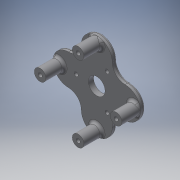
# Autodesk Inventor part: cycloid_motor_fix_plate
Saved by Autodesk Inventor 2019.4 (Build 234330000, 330)
## iProperties
Created: 2019-08-28
Part Number: cycloid_motor_fix_plate
Material: Generic
Document SubType Name: Modeling
Designer: cdi
Density: 1 g/cm^3
Appearance: Default
Author: cdi
Autodesk Inventor part; units mm, degrees
ref_plane "YZ Plane" through (0, 0, 0) normal (1, 0, 0) x (0, 1, 0)
ref_plane "XZ Plane" through (0, 0, 0) normal (0, 1, 0) x (-1, 0, 0)
ref_plane "XY Plane" through (0, 0, 0) normal (0, 0, 1) x (1, 0, 0)
sketch "Sketch1" plane through (0, 0, 0) normal (0, 0, 1) x (1, 0, 0)
  circle A0 centre (0, 0) radius 34
  dimension "d2" = 68
  constraints: 1 centre point, 1 coincident
  measures "d2" diameter of A0
extrude "Extrusion1" add sketch "Sketch1" along normal blind 4
sketch "Sketch3" plane through (0, 0, 0) normal (0, 0, -1) x (-1, 0, 0)
  circle A0 centre (0, 0) radius 6.5
  dimension "d15" = 13
  constraints: 1 centre point, 1 coincident
  measures "d15" diameter of A0
extrude "Extrusion2" cut sketch "Sketch3" against normal through all
sketch "Sketch4" plane through (0, 0, 0) normal (0, 0, -1) x (-1, 0, 0)
  circle A0 centre (0, 0) radius 9.5
  circle A1 centre (0, 9.5) radius 1.5
  circle A2 centre (-6.7175, 6.7175) radius 1.5
  circle A3 centre (-9.5, 0) radius 1.5
  circle A4 centre (-6.7175, -6.7175) radius 1.5
  circle A5 centre (0, -9.5) radius 1.5
  circle A6 centre (6.7175, -6.7175) radius 1.5
  circle A7 centre (9.5, 0) radius 1.5
  circle A8 centre (6.7175, 6.7175) radius 1.5
  circle A9 centre (0, 0) radius 16
  circle A10 centre (16, 0) radius 1.5
  circle A11 centre (-8, 13.8564) radius 1.5
  circle A12 centre (-8, -13.8564) radius 1.5
  point P0 (-6.9376, -6.7295)
  dimension "d18" = 19
  dimension "d24" = 32
  dimension "d19" = 3
  dimension "d22" = 360
  dimension "d25" = 3
  dimension "d28" = 360
  constraints: 11 centre point, 2 coincident, 1 horizontal alignment, 1 vertical alignment, 28 other
  measures "d19" diameter of A1
  measures "d25" diameter of A10
hole "Hole2" at (8, 13.8564, 0) at (-16, 0, 0) at (8, -13.8564, 0) direction (0, 0, 1) diameter 3.1 depth 10 countersink diameter 6.5 countersink angle 90
sketch "Sketch5" plane through (0, 0, 4) normal (0, 0, 1) x (1, 0, 0)
  line L0 (-80.396, -12) -> (-12, -12)
  line L1 (-12, -12) -> (-12, -63.9802)
  line L2 (-12, -63.9802) -> (-80.396, -63.9802)
  line L3 (-80.396, -63.9802) -> (-80.396, -12)
  line L4 (0, 0) -> (-93.0099, 0)
  line L5 (0, 0) -> (0, -83.9307)
  dimension "d37" = 12
  dimension "d38" = 12
  constraints: 12 end point, 2 horizontal, 2 parallel, 1 perpendicular, 1 vertical
  measures "d37" distance between parallel lines of L1 L5
  measures "d38" distance between parallel lines of L4 L0
extrude "Extrusion3" cut sketch "Sketch5" against normal through all
pattern_circular "Circular Pattern2" count 4 over 360 about axis through (0, 0, 0) along (0, 0, 1) of "Extrusion3"
fillet "Fillet1" radius 10 4 edges at (-12, -12, 2) (12, 12, 2) (-12, 12, 2) (12, -12, 2)
fillet "Fillet1" radius 12 8 edges at (12, 31.8119, 2) (-12, 31.8119, 2) (-31.8119, 12, 2) (-31.8119, -12, 2) (-12, -31.8119, 2) (12, -31.8119, 2) (31.8119, -12, 2) (31.8119, 12, 2)
sketch "Sketch6" plane through (0, 0, 4) normal (0, 0, 1) x (1, 0, 0)
  circle A0 centre (0, 29.5) radius 1.625 projected
  circle A1 centre (0, 29.5) radius 4.5
  point P0 (0, 0)
  dimension "d46" = 9
  constraints: 1 centre point, 1 coincident
  measures "d46" diameter of A1
extrude "Extrusion4" add sketch "Sketch6" along normal blind 14.5
pattern_circular "Circular Pattern3" count 4 over 360 about axis through (0, 0, 0) along (0, 0, 1) of "Extrusion4"
fillet "Fillet3" radius 2 12 edges at (-3.1819, 26.318, 4) (3.182, 32.6819, 4) (0, 34, 4) (-26.318, -3.1819, 4) (-32.6819, 3.182, 4) (-34, 0, 4) (3.1819, -26.318, 4) (-3.182, -32.6819, 4) (0, -34, 4) (32.6819, -3.182, 4) (34, 0, 4) (26.318, 3.1819, 4)
fillet "Fillet4" radius 2 24 edges at (-12, -22, 0) (-14.9289, -14.9289, 0) (-22, -12, 0) (12, -22, 0) (8.4853, -30.4853, 0) (-8.4853, -30.4853, 0) (0, -34, 0) (22, -12, 0) (14.9289, -14.9289, 0) (30.4853, 8.4853, 0) (22, 12, 0) (30.4853, -8.4853, 0) (34, 0, 0) (12, 22, 0) (14.9289, 14.9289, 0) (-12, 22, 0) (-8.4853, 30.4853, 0) (8.4853, 30.4853, 0) (0, 34, 0) (-22, 12, 0) (-14.9289, 14.9289, 0) (-30.4853, 8.4853, 0) (-30.4853, -8.4853, 0) (-34, 0, 0)
sketch "Sketch2" plane through (0, 0, 0) normal (0, 0, -1) x (-1, 0, 0)
  circle A0 centre (0, 29.5) radius 3.5
  point P0 (0, 0)
  dimension "d3" = 7
  dimension "d4" = 29.5
  constraints: 1 centre point
  measures "d3" diameter of A0
  measures "d4" distance of point (0, 0) A0.centre
extrude "Extrusion5" cut sketch "Sketch2" against normal blind 3
sketch "Sketch9" plane through (0, 29.5, 3) normal (0, 0, -1) x (-1, 0, 0)
  arc A0 (-2.8, 2.1) -> (2.8, 2.1) centre (0, 0) ccw projected
  point P0 (0, -29.5)
hole "Hole5" at (0, 29.5, 3) direction (0, 0, 1) diameter 3.25 depth 15 countersink diameter 6.5 countersink angle 90
fillet "Fillet6" radius 0.4 5 edges at (1.5811, 32.6225, 0.1417) (-1.5811, 32.6225, 0.1417) (0, 33, 0.2679) (-3.3204, 30.6068, 0) (1.1068, 26.1796, 0)
pattern_circular "Circular Pattern5" count 4 over 360 about axis through (0, 0, 0) along (0, 0, 1) of "Extrusion5", "Hole5", "Fillet6"
body "Solid1"
